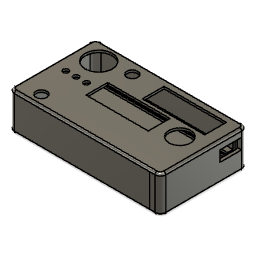
Full Case v1 (Autodesk Fusion 360 design; units mm, degrees)
Autodesk Fusion 360 part; units mm, degrees
note: some values were not read from the file. Chosen so that the rebuilt part matches the saved one: which bodies a step acts on; which face or edge a step refers to.
sketch "Sketch1" plane through (0, 0, 0) normal (0, 1, 0) x (1, 0, 0)
  line L0 (6.35, 0) -> (171.45, 0)
  line L1 (177.8, 6.35) -> (177.8, 95.25)
  line L2 (171.45, 101.6) -> (6.35, 101.6)
  line L3 (0, 95.25) -> (0, 6.35)
  arc A0 (177.8, 95.25) -> (171.45, 101.6) centre (171.45, 95.25) ccw
  arc A1 (6.35, 101.6) -> (0, 95.25) centre (6.35, 95.25) ccw
  arc A2 (0, 6.35) -> (6.35, 0) centre (6.35, 6.35) ccw
  arc A3 (171.45, 0) -> (177.8, 6.35) centre (171.45, 6.35) ccw
  point P0 (177.8, 0)
  point P1 (177.8, 101.6)
  dimension "length" = 177.8
  dimension "width" = 101.6
  dimension "d3" = 6.35
  constraint horizontal L0
  constraint vertical L1
  constraint horizontal L2
  constraint vertical L3
  constraint coincident P1 L1
  constraint coincident P1 L2
  constraint tangent L1 A0
  constraint tangent L2 A0
  constraint tangent L2 A1
  constraint tangent L3 A1
  constraint equal A0 A1
  constraint coincident origin L0
  constraint coincident origin L3
  constraint tangent L0 A2
  constraint tangent L3 A2
  constraint equal A0 A2
  constraint coincident P0 L0
  constraint coincident P0 L1
  constraint tangent L0 A3
  constraint tangent L1 A3
  constraint equal A0 A3
  measures "length" distance of origin P0
  measures "width" distance of P0 P1
  measures "d3" radius of A0
extrude "Extrude1" add sketch "Sketch1" along normal blind 2.54 makes body 1
sketch "Sketch2" plane through (0, 2.54, 0) normal (0, 1, 0) x (-1, 0, 0)
  arc A0 (-171.45, 0) -> (-177.8, -6.35) centre (-171.45, -6.35) ccw
  line L0 (-177.8, -6.35) -> (-177.8, -95.25)
  arc A1 (-177.8, -95.25) -> (-171.45, -101.6) centre (-171.45, -95.25) ccw
  line L1 (-171.45, -101.6) -> (-6.35, -101.6)
  arc A2 (-6.35, -101.6) -> (0, -95.25) centre (-6.35, -95.25) ccw
  line L2 (0, -95.25) -> (0, -6.35)
  arc A3 (0, -6.35) -> (-6.35, 0) centre (-6.35, -6.35) ccw
  line L3 (-6.35, 0) -> (-171.45, 0)
  line L4 (-10.16, -97.79) -> (-167.64, -97.79)
  line L5 (-173.99, -91.44) -> (-173.99, -10.16)
  line L6 (-167.64, -3.81) -> (-10.16, -3.81)
  line L7 (-3.81, -10.16) -> (-3.81, -91.44)
  arc A4 (-10.16, -97.79) -> (-3.81, -91.44) centre (-10.16, -91.44) ccw
  arc A5 (-3.81, -10.16) -> (-10.16, -3.81) centre (-10.16, -10.16) ccw
  arc A6 (-167.64, -3.81) -> (-173.99, -10.16) centre (-167.64, -10.16) ccw
  arc A7 (-173.99, -91.44) -> (-167.64, -97.79) centre (-167.64, -91.44) ccw
  dimension "d8" = 6.35
  dimension "d12" = 3.81
  dimension "d14" = 3.81
  dimension "d15" = 3.81
  dimension "d17" = 3.81
  constraint horizontal L4
  constraint vertical L5
  constraint horizontal L6
  constraint vertical L7
  constraint tangent L4 A4
  constraint tangent L7 A4
  constraint tangent L6 A5
  constraint tangent L7 A5
  constraint equal A4 A5
  constraint tangent L5 A6
  constraint tangent L6 A6
  constraint equal A4 A6
  constraint tangent L4 A7
  constraint tangent L5 A7
  constraint equal A4 A7
  measures "d8" radius of A4
  measures "d12" distance of L2 L7
  measures "d14" distance of L1 L4
  measures "d15" distance of L3 L6
  measures "d17" distance of L0 L5
extrude "Extrude3" add sketch "Sketch2" along normal blind 38.1 separate body makes body 2
sketch "Sketch3" plane through (0, 40.64, 0) normal (0, 1, 0) x (-1, 0, 0)
  arc A0 (-167.64, -3.81) -> (-173.99, -10.16) centre (-167.64, -10.16) ccw
  line L0 (-167.64, -3.81) -> (-10.16, -3.81)
  arc A1 (-3.81, -10.16) -> (-10.16, -3.81) centre (-10.16, -10.16) ccw
  line L1 (-3.81, -10.16) -> (-3.81, -91.44)
  arc A2 (-10.16, -97.79) -> (-3.81, -91.44) centre (-10.16, -91.44) ccw
  line L2 (-10.16, -97.79) -> (-167.64, -97.79)
  arc A3 (-173.99, -91.44) -> (-167.64, -97.79) centre (-167.64, -91.44) ccw
  line L3 (-173.99, -91.44) -> (-173.99, -10.16)
  line L4 (-6.35, 0) -> (-171.45, 0)
  arc A4 (-171.45, 0) -> (-177.8, -6.35) centre (-171.45, -6.35) ccw
  line L5 (-177.8, -6.35) -> (-177.8, -95.25)
  arc A5 (-177.8, -95.25) -> (-171.45, -101.6) centre (-171.45, -95.25) ccw
  line L6 (-171.45, -101.6) -> (-6.35, -101.6)
  arc A6 (-6.35, -101.6) -> (0, -95.25) centre (-6.35, -95.25) ccw
  line L7 (0, -95.25) -> (0, -6.35)
  arc A7 (0, -6.35) -> (-6.35, 0) centre (-6.35, -6.35) ccw
  line L8 (-6.35, -101.6) -> (-171.45, -101.6)
  line L9 (-177.8, -95.25) -> (-177.8, -6.35)
  line L10 (-171.45, 0) -> (-6.35, 0)
  line L11 (0, -6.35) -> (0, -95.25)
  arc A8 (-6.35, -101.6) -> (0, -95.25) centre (-6.35, -95.25) ccw
  arc A9 (0, -6.35) -> (-6.35, 0) centre (-6.35, -6.35) ccw
  arc A10 (-171.45, 0) -> (-177.8, -6.35) centre (-171.45, -6.35) ccw
  arc A11 (-177.8, -95.25) -> (-171.45, -101.6) centre (-171.45, -95.25) ccw
  line L12 (-52.3875, -63.5) -> (-125.4125, -63.5)
  line L13 (-125.4125, -63.5) -> (-125.4125, -38.1)
  line L14 (-125.4125, -38.1) -> (-52.3875, -38.1)
  line L15 (-52.3875, -38.1) -> (-52.3875, -63.5)
  circle A12 centre (-149.7013, -50.8) radius 12.7
  circle A13 centre (-15.9544, -50.8) radius 3.175
  circle A14 centre (-28.0987, -50.8) radius 3.175
  circle A15 centre (-40.2431, -50.8) radius 3.175
  line L16 (-89.3763, -92.71) -> (-162.4013, -92.71)
  line L17 (-162.4013, -92.71) -> (-162.4013, -67.31)
  line L18 (-162.4013, -67.31) -> (-89.3763, -67.31)
  line L19 (-89.3763, -67.31) -> (-89.3763, -92.71)
  line L20 (-149.7013, -50.8) -> (-125.4125, -50.8)
  line L21 (-149.7013, -50.8) -> (-173.99, -50.8)
  line L22 (-3.81, -50.8) -> (-15.9544, -50.8)
  line L23 (-15.9544, -50.8) -> (-28.0987, -50.8)
  line L24 (-40.2431, -50.8) -> (-52.3875, -50.8)
  line L25 (-28.0987, -50.8) -> (-40.2431, -50.8)
  circle A16 centre (-58.42, -86.36) radius 6.35
  circle A17 centre (-25.4, -12.7) radius 6.35
  circle A18 centre (-25.4, -80.01) radius 15.875
  point P0 (-3.81, -50.8)
  point P1 (-52.3875, -50.8)
  point P2 (-88.9, -63.5)
  point P3 (-88.9, -97.79)
  point P4 (-173.99, -50.8)
  point P5 (-89.3763, -80.01)
  dimension "d19" = 6.35
  dimension "d20" = 73.025
  dimension "d21" = 25.4
  dimension "d23" = 6.35
  dimension "d29" = 5.08
  dimension "d31" = 25.4
  dimension "d34" = 12.7
  dimension "d35" = 12.7
  dimension "d39" = 31.75
  constraint horizontal L8
  constraint vertical L9
  constraint horizontal L10
  constraint vertical L11
  constraint tangent L8 A8
  constraint tangent L11 A8
  constraint tangent L10 A9
  constraint tangent L11 A9
  constraint equal A8 A9
  constraint tangent L9 A10
  constraint tangent L10 A10
  constraint equal A8 A10
  constraint tangent L8 A11
  constraint tangent L9 A11
  constraint equal A8 A11
  constraint horizontal L12
  constraint vertical L13
  constraint horizontal L14
  constraint vertical L15
  constraint equal L4 L10
  constraint equal L5 L9
  constraint collinear L6 L8
  constraint collinear L5 L9
  constraint midpoint L1 P0
  constraint midpoint L15 P1
  constraint horizontal P0 P1
  constraint midpoint L12 P2
  constraint midpoint L2 P3
  constraint vertical P2 P3
  constraint equal A13 A14
  constraint equal A13 A15
  constraint horizontal L16
  constraint vertical L17
  constraint horizontal L18
  constraint vertical L19
  constraint equal L12 L16
  constraint equal L15 L19
  constraint horizontal P0 A13.centre
  constraint horizontal A13.centre A14.centre
  constraint horizontal A14.centre A15.centre
  constraint midpoint L3 P4
  constraint horizontal A12.centre P4
  constraint coincident A12.centre L20.start
  constraint midpoint L13 L20.end
  constraint perpendicular L13 L20
  constraint coincident P4 L21.end
  constraint perpendicular L3 L21
  constraint equal L20 L21
  constraint coincident P0 L22.start
  constraint coincident A13.centre L22.end
  constraint perpendicular L1 L22
  constraint coincident A14.centre L23.end
  constraint coincident A15.centre L24.start
  constraint coincident P1 L24.end
  constraint perpendicular L15 L24
  constraint equal L24 L25
  constraint equal L23 L25
  constraint equal L22 L23
  constraint midpoint L19 P5
  constraint horizontal A18.centre P5
  constraint vertical A17.centre A18.centre
  constraint tangent L16 A16
  constraint tangent A12 L17
  measures "d19" radius of A8
  measures "d20" distance of L12.start L12.end
  measures "d21" distance of L12.start L14.end
  measures "d23" diameter of A13
  measures "d29" distance of L2 L16
  measures "d31" diameter of A12
  measures "d34" diameter of A16
  measures "d35" diameter of A17
  measures "d39" diameter of A18
extrude "Extrude4" add sketch "Sketch3" along normal blind 2.54 separate body contours A0 L0 A1 L1 L3 L13 L14 L15 A12 A13 A14 A15 L20 L21 L22 L23 L24 L25 | L1 A2 L2 A3 L3 L12 L13 L15 A12 A13 A14 A15 L20 L21 L22 L23 L24 L25 | L4 A4 L5 A5 L6 A6 L7 A7 L8 L9 L10 L11 A8 A9 A10 A11 makes body 3
sketch "Sketch4" plane through (177.8, 0, 0) normal (1, 0, 0) x (0, 0, -1)
  line L0 (6.35, 2.54) -> (95.25, 2.54)
  line L1 (95.25, 2.54) -> (95.25, 40.64)
  line L2 (95.25, 40.64) -> (6.35, 40.64)
  line L3 (6.35, 40.64) -> (6.35, 2.54)
  line L4 (95.25, 34.29) -> (69.85, 34.29)
  line L5 (69.85, 34.29) -> (69.85, 21.59)
  line L6 (69.85, 21.59) -> (95.25, 21.59)
  line L7 (95.25, 21.59) -> (95.25, 34.29)
  line L8 (0, 2.54) -> (101.6, 2.54)
  line L9 (0, 40.64) -> (101.6, 40.64)
  line L10 (6.35, 43.18) -> (95.25, 43.18)
  line L11 (6.35, 0) -> (95.25, 0)
  dimension "d36" = 12.7
  dimension "d49" = 25.4
  dimension "d50" = 6.35
  dimension "d51" = 101.6
  dimension "d52" = 101.6
  dimension "trimD" = 2.54
  dimension "d54" = 2.54
  constraint horizontal L4
  constraint vertical L5
  constraint horizontal L6
  constraint vertical L7
  constraint coincident L1 L4.start
  constraint perpendicular L1 L8
  constraint perpendicular L1 L9
  measures "d36" distance of L4.start L6.end
  measures "d49" distance of L4.start L4.end
  measures "d50" distance of L2 L4
  measures "d51" distance of L8.start L8.end
  measures "d52" distance of L9.start L9.end
  measures "trimD" distance of L9 L10
  measures "d54" distance of L8 L11
extrude "Extrude5" cut sketch "Sketch4" against normal blind 12.7 contours L1 L4 L5 L6 L7 bodies 2
sketch "Sketch5" plane through (0, 43.18, 0) normal (0, 1, 0) x (-1, 0, 0)
  circle A0 centre (-15.9544, -50.8) radius 3.175
  circle A1 centre (-28.0987, -50.8) radius 3.175
  circle A2 centre (-40.2431, -50.8) radius 3.175
  line L0 (-162.4013, -67.31) -> (-89.3763, -67.31)
  line L1 (-89.3763, -67.31) -> (-89.3763, -92.71)
  line L2 (-89.3763, -92.71) -> (-162.4013, -92.71)
  line L3 (-162.4013, -92.71) -> (-162.4013, -67.31)
  circle A3 centre (-58.42, -86.36) radius 6.35
  circle A4 centre (-25.4, -80.01) radius 15.875
  circle A5 centre (-25.4, -12.7) radius 6.35
  circle A6 centre (-149.7013, -50.8) radius 12.7
  line L4 (-125.4125, -38.1) -> (-52.3875, -38.1)
  line L5 (-52.3875, -38.1) -> (-52.3875, -63.5)
  line L6 (-52.3875, -63.5) -> (-125.4125, -63.5)
  line L7 (-125.4125, -63.5) -> (-125.4125, -38.1)
  line L8 (-165.1, -101.6) -> (-165.1, 0)
  arc A7 (-171.45, 0) -> (-177.8, -6.35) centre (-171.45, -6.35) ccw
  line L9 (-177.8, -6.35) -> (-177.8, -95.25)
  arc A8 (-177.8, -95.25) -> (-171.45, -101.6) centre (-171.45, -95.25) ccw
  line L10 (-171.45, -101.6) -> (-6.35, -101.6)
  arc A9 (-6.35, -101.6) -> (0, -95.25) centre (-6.35, -95.25) ccw
  line L11 (0, -95.25) -> (0, -6.35)
  arc A10 (0, -6.35) -> (-6.35, 0) centre (-6.35, -6.35) ccw
  line L12 (-6.35, 0) -> (-171.45, 0)
  point P0 (-165.1, -50.8)
  point P1 (-173.4006, -50.8)
  dimension "d44" = 101.6
  constraint vertical L8
  constraint midpoint L8 P0
  constraint horizontal P0 P1
  measures "d44" distance of L8.start L8.end
split "Split1" by curves path "Sketch5" along L8 bodies 1 2 3 makes body 6 at (107.053, 40.64, -15.741) makes body 5 at (112.1833, 27.94, 0) makes body 4 at (112.1833, 0, -33.8667)
combine "Combine1" operation add target body 1 tool bodies 2 3
split "Split2" by curves path "Sketch4" along L9 L8 bodies 1 makes body 7 at (177.8, 21.59, -27.5167) makes body 8 at (169.3333, 0, -35.9833)
combine "Combine2" operation add target body 6 tool bodies 1
combine "Combine3" operation add target body 4 tool bodies 8
fillet "Fillet3" radius 2.54 8 edges at (88.9, 43.18, -101.6) (1.8599, 43.18, -99.7401) (0, 43.18, -50.8) (1.8599, 43.18, -1.8599) (88.9, 43.18, 0) (175.9401, 43.18, -1.8599) (177.8, 43.18, -50.8) (175.9401, 43.18, -99.7401) on bodies 6
fillet "Fillet4" radius 2.54 8 edges at (88.9, 0, -101.6) (1.8599, 0, -99.7401) (0, 0, -50.8) (1.8599, 0, -1.8599) (88.9, 0, 0) (175.9401, 0, -1.8599) (177.8, 0, -50.8) (175.9401, 0, -99.7401) on bodies 4
sketch "Sketch13" plane through (165.1, 0, 0) normal (1, 0, 0) x (0, 0, -1)
  line L0 (101.6, 2.54) -> (101.6, 40.64)
  line L1 (101.6, 40.64) -> (97.79, 40.64)
  line L2 (97.79, 40.64) -> (97.79, 2.54)
  line L3 (97.79, 2.54) -> (101.6, 2.54)
  line L4 (97.79, 40.64) -> (3.81, 40.64)
  line L5 (3.81, 40.64) -> (3.81, 2.54)
  line L6 (3.81, 2.54) -> (97.79, 2.54)
  line L7 (97.79, 2.54) -> (97.79, 40.64)
  line L8 (3.81, 7.62) -> (10.16, 7.62)
  line L9 (10.16, 7.62) -> (10.16, 10.16)
  line L10 (10.16, 10.16) -> (3.81, 10.16)
  line L11 (3.81, 10.16) -> (3.81, 7.62)
  line L12 (3.81, 11.811) -> (10.16, 11.811)
  line L13 (10.16, 11.811) -> (10.16, 14.351)
  line L14 (10.16, 14.351) -> (3.81, 14.351)
  line L15 (3.81, 14.351) -> (3.81, 11.811)
  line L16 (50.8, 40.64) -> (50.8, 2.54)
  line L17 (97.79, 14.351) -> (97.79, 11.811)
  line L18 (91.44, 10.16) -> (97.79, 10.16)
  line L19 (97.79, 7.62) -> (91.44, 7.62)
  line L20 (91.44, 7.62) -> (91.44, 10.16)
  line L21 (91.44, 14.351) -> (97.79, 14.351)
  line L22 (91.44, 11.811) -> (91.44, 14.351)
  line L23 (97.79, 11.811) -> (91.44, 11.811)
  line L24 (97.79, 10.16) -> (97.79, 7.62)
  line L25 (10.16, 2.54) -> (10.16, 40.64)
  dimension "d57" = 93.98
  dimension "d58" = 38.1
  dimension "d59" = 6.35
  dimension "d60" = 2.54
  dimension "d61" = 6.35
  dimension "d62" = 2.54
  dimension "bThick" = 1.651
  dimension "d64" = 5.08
  constraint horizontal L4
  constraint vertical L5
  constraint horizontal L6
  constraint vertical L7
  constraint coincident L1.end L2.start
  constraint horizontal L8
  constraint vertical L9
  constraint horizontal L10
  constraint vertical L11
  constraint horizontal L12
  constraint vertical L13
  constraint horizontal L14
  constraint vertical L15
  constraint midpoint L4 L16.start
  constraint midpoint L6 L16.end
  constraint symmetric L8.start L16 L19.start
  constraint symmetric L8.end L16 L19.end
  constraint symmetric L9.end L16 L18.start
  constraint symmetric L10.end L16 L18.end
  constraint symmetric L12.start L16 L17.end
  constraint symmetric L12.end L16 L22.start
  constraint symmetric L13.end L16 L21.start
  constraint symmetric L14.end L16 L17.start
  constraint collinear L11 L15
  constraint collinear L5 L11
  measures "d57" distance of L1.end L4.end
  measures "d58" distance of L4.end L5.end
  measures "d59" distance of L8.start L8.end
  measures "d60" distance of L8.start L10.end
  measures "d61" distance of L12.start L12.end
  measures "d62" distance of L12.start L14.end
  measures "bThick" distance of L10 L12
  measures "d64" distance of L6 L8
extrude "Extrude6" add sketch "Sketch13" against normal up to surface (161.29 mm away) contours L2 L7 L18 L19 L20 L24 | L2 L7 L17 L21 L22 L23 | L5 L8 L9 L10 L11 L25 | L5 L12 L13 L14 L15 L25 bodies 5
equation "d23 = ( 1 / 4 ) * 1 in"
equation "buttonD = 0.5 in"
equation "joystickDbuttonD = 0.7 in"
equation "d34 = ( 1 / 2 ) * 1 in"
equation "d35 = ( 1 / 2 ) * 1 in"
equation "d36 = ( 1 / 2 ) * 1 in"
equation "d44 = width"
equation "d51 = width"
equation "d52 = width"
equation "d54 = trimD"
equation "d57 = width - 0.3 in"
equation "d59 = ( 1 / 4 ) * 1 in"
named bodies: "Side(1)", "Bottom", "Walls", "Top", "Side", "Side (2)"
